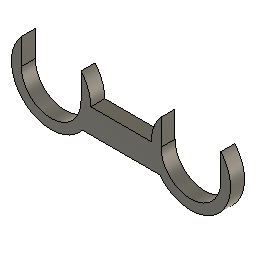
saddle_coupon (Autodesk Fusion 360 design; units mm, degrees)
part number: 2026-09-02-15-19-08-139
Autodesk Fusion 360 part; units mm, degrees
sketch "Coupon chord" plane through (0, 0, 0) normal (0, 1, 0) x (1, 0, 0)
  line L0 (70, -62) -> (150, -62)
  line L1 (150, -62) -> (150, -76)
  line L2 (150, -76) -> (70, -76)
  line L3 (70, -76) -> (70, -62)
extrude "Coupon chord (1)" add sketch "Coupon chord" along normal mid plane 8
sketch "Saddle boss x=70" plane through (0, 0, 0) normal (0, 1, 0) x (1, 0, 0)
  circle A0 centre (70, -76) radius 22.7
extrude "Saddle boss x=70 (1)" add sketch "Saddle boss x=70" along normal mid plane 8
sketch "Saddle boss x=150" plane through (0, 0, 0) normal (0, 1, 0) x (1, 0, 0)
  circle A0 centre (150, -76) radius 22.7
extrude "Saddle boss x=150 (1)" add sketch "Saddle boss x=150" along normal mid plane 8
sketch "Rod pocket x=70" plane through (0, 0, 0) normal (0, 1, 0) x (1, 0, 0)
  circle A0 centre (70, -76) radius 17.1
extrude "Rod pocket x=70 (1)" cut sketch "Rod pocket x=70" along normal mid plane 18
sketch "Drop-in opening x=70" plane through (0, 0, 0) normal (0, 1, 0) x (1, 0, 0)
  line L0 (52.9, -76) -> (87.1, -76)
  line L1 (87.1, -76) -> (87.1, -103.7)
  line L2 (87.1, -103.7) -> (52.9, -103.7)
  line L3 (52.9, -103.7) -> (52.9, -76)
extrude "Drop-in opening x=70 (1)" cut sketch "Drop-in opening x=70" along normal mid plane 18
sketch "Rod pocket x=150" plane through (0, 0, 0) normal (0, 1, 0) x (1, 0, 0)
  circle A0 centre (150, -76) radius 17.1
extrude "Rod pocket x=150 (1)" cut sketch "Rod pocket x=150" along normal mid plane 18
sketch "Drop-in opening x=150" plane through (0, 0, 0) normal (0, 1, 0) x (1, 0, 0)
  line L0 (132.9, -76) -> (167.1, -76)
  line L1 (167.1, -76) -> (167.1, -103.7)
  line L2 (167.1, -103.7) -> (132.9, -103.7)
  line L3 (132.9, -103.7) -> (132.9, -76)
extrude "Drop-in opening x=150 (1)" cut sketch "Drop-in opening x=150" along normal mid plane 18
named bodies: "saddle_coupon"
